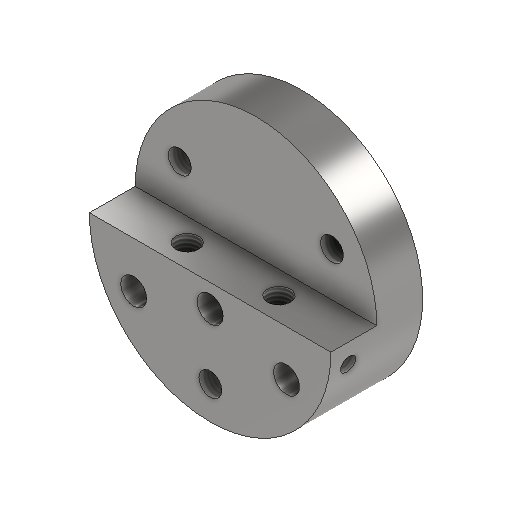
# Autodesk Inventor part: B_probehead_5_1
Saved by Autodesk Inventor 2026.2 (Build 302298000, 298)
## iProperties
Created: 2026-02-02
Part Number: B_probehead_5_1
Material: ステンレス鋼 440C
Document SubType Name: Modeling
Designer: zetsu
Density: 7.75 g/cm^3
Appearance: 半つや出し
Author: zetsu
Autodesk Inventor part; units mm, degrees
ref_plane "XZ Plane" through (0, 0, 0) normal (0, 1, 0) x (-1, 0, 0)
sketch "スケッチ2" plane through (0, 0, 0) normal (0, 0, 1) x (1, 0, 0)
  circle A0 centre (0, 0) radius 15.8
  dimension "d0" = 31.6
  constraints: 1 centre point, 1 coincident
  measures "d0" diameter of A0
extrude "押し出し1" add sketch "スケッチ2" against normal blind 12
sketch "スケッチ4" plane through (0, 0, 0) normal (0, 0, 1) x (1, 0, 0)
  circle A0 centre (0.0258, -11.5) radius 1.5
  circle A1 centre (9.9464, 5.7723) radius 1.5
  circle A2 centre (-9.9722, 5.7277) radius 1.5
  point P0 (0, 0)
  dimension "d8" = 3
  dimension "d9" = 11.5
  dimension "d12" = 360
  constraints: 3 centre point, 7 other
  measures "d8" diameter of A0
  measures "d9" distance of A0.centre point (0, 0)
extrude "押し出し3" cut sketch "スケッチ4" against normal through all
sketch "スケッチ13" plane through (0, 0, 0) normal (0, 0, 1) x (1, 0, 0)
  circle A0 centre (-10, -6) radius 1.7
  circle A1 centre (10, -6) radius 1.7
  circle A2 centre (0, -3) radius 1.7
  line L0 (0, 0) -> (0, -19.4065)
  line L1 (0, 0) -> (20.4623, 0)
  point P0 (0, -4.7)
  point P1 (0, -1.3)
  dimension "d125" = 3.4
  dimension "d126" = 3.4
  dimension "d127" = 3.4
  dimension "d128" = 6
  dimension "d129" = 3
  dimension "d130" = 10
  constraints: 4 end point, 3 centre point, 1 horizontal, 1 symmetric about line, 1 vertical
  measures "d125" diameter of A0
  measures "d126" diameter of A1
  measures "d127" diameter of A2
  measures "d128" vertical distance of L0.start A1.centre
  measures "d129" distance of A2.centre L0.start
  measures "d130" horizontal distance of A1.centre L0.start
extrude "押し出し11" cut sketch "スケッチ13" against normal through all
ref_plane "作業平面6" through (0, 0, 0) normal (0.9848, -0.1736, 0) x (0, 0, 1)
ref_plane "作業平面7" through (0, 0, 0) normal (0.9848, 0.1736, 0) x (0, 0, 1)
ref_plane "作業平面8" through (15.56, -2.7436, 0) normal (0.9848, -0.1736, 0) x (0, 0, 1)
ref_plane "作業平面9" through (-15.56, -2.7436, 0) normal (0.9848, 0.1736, 0) x (0, 0, 1)
sketch "スケッチ15" plane through (15.56, -2.7436, 0) normal (0.9848, -0.1736, 0) x (0, 0, 1)
  circle A0 centre (-2.5, 0) radius 1
  point P0 (0, 0)
  dimension "d103" = 2
  dimension "d104" = 2.5
  constraints: 1 centre point
  measures "d103" diameter of A0
  measures "d104" distance of A0.centre point (0, 0)
sketch "スケッチ16" plane through (-15.56, -2.7436, 0) normal (0.9848, 0.1736, 0) x (0, 0, 1)
  circle A0 centre (-2.5, 0) radius 1
  point P0 (0, 0)
  dimension "d105" = 2
  dimension "d106" = 2.5
  constraints: 1 centre point
  measures "d105" diameter of A0
  measures "d106" distance of point (0, 0) A0.centre
extrude "押し出し12" cut sketch "スケッチ16" along normal blind 6
extrude "押し出し13" cut sketch "スケッチ15" against normal blind 6
thread "ねじ10" size "M2x0.4" class "6H" standard "ANSI Metric M Profile" full length
thread "ねじ11" size "M2x0.4" class "6H" standard "ANSI Metric M Profile" full length
sketch "スケッチ18" plane through (0, 0, 0) normal (0, 0, 1) x (1, 0, 0)
  line L0 (-18.9802, 17.2113) -> (19.0758, 17.2113)
  line L1 (19.0758, 17.2113) -> (19.0758, 0)
  line L2 (19.0758, 0) -> (-18.9802, 0)
  line L3 (-18.9802, 0) -> (-18.9802, 17.2113)
  point P0 (0, 0)
  point P1 (0.0478, 0)
  dimension "d141" = 0
  constraints: 8 end point, 2 parallel, 1 horizontal, 1 midpoint, 1 perpendicular
  measures "d141" distance from line of point (0, 0) L2
extrude "押し出し15" cut sketch "スケッチ18" against normal blind 6
sketch "スケッチ20" plane through (-15.8, 0, 0) normal (0, 1, 0) x (1, 0, 0)
  line L0 (15.8, 0) -> (15.8, 8.7821) construction
  line L1 (0, 0) -> (0, 6) projected
  line L2 (0, 3) -> (33.9854, 3) construction
  circle A0 centre (9.8, 3) radius 1.5
  circle A1 centre (21.8, 3) radius 1.5
  line L3 (31.6, 0) -> (0, 0) projected
  dimension "d132" = 3
  dimension "d133" = 3
  dimension "d134" = 6
  constraints: 4 end point, 2 centre point, 2 midpoint, 2 point on line, 1 symmetric about line, 1 vertical
  measures "d132" diameter of A0
  measures "d133" diameter of A1
  measures "d134" horizontal distance of point (15.8, 0) A1.centre
extrude "押し出し16" cut sketch "スケッチ20" against normal blind 8
thread "ねじ13" size "M3x0.5" class "6H" standard "ANSI Metric M Profile" full length
thread "ねじ14" size "M3x0.5" class "6H" standard "ANSI Metric M Profile" full length
thread "ねじ15" size "M3x0.5" class "6H" standard "ANSI Metric M Profile" full length
thread "ねじ16" size "M3x0.5" class "6H" standard "ANSI Metric M Profile" full length
thread "ねじ17" size "M3x0.5" class "6H" standard "ANSI Metric M Profile" full length
